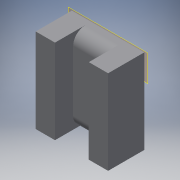
# Autodesk Inventor part: commutator_attachement_side_plate
Saved by Autodesk Inventor 2016 (Build 200138000, 138)
## iProperties
Created: 2016-09-28
Part Number: commutator_attachement_side_plate
Material: Generic
Document SubType Name: Modeling
Designer: ajar021
Density: 1 g/cm^3
Appearance: Default
Author: ajar021
Autodesk Inventor part; units mm, degrees
ref_plane "YZ Plane" through (0, 0, 0) normal (1, 0, 0) x (0, 1, 0)
ref_plane "XZ Plane" through (0, 0, 0) normal (0, 1, 0) x (-1, 0, 0)
ref_plane "XY Plane" through (0, 0, 0) normal (0, 0, 1) x (1, 0, 0)
ref_plane "Work Plane1" through (0, 0, 0) normal (0, 0, 1) x (1, 0, 0)
sketch "Sketch1" plane through (0, 0, 0) normal (0, 0, 1) x (1, 0, 0)
  line L0 (12, 0) -> (12, 4) projected
  line L1 (0, 4) -> (12, 4) projected
  line L2 (0, 0) -> (0, 4) projected
  line L3 (12, 0) -> (12, -10)
  line L4 (12, -10) -> (0, -10)
  line L5 (0, -10) -> (0, 4)
  line L6 (0, 4) -> (12, 4)
  line L7 (12, 4) -> (12, 0)
  dimension "d0" = 10
  constraints: 10 end point, 3 collinear, 1 perpendicular, 1 vertical
  measures "d0" distance of L0.start L3.end
extrude "Extrusion1" add sketch "Sketch1" along normal blind 3
sketch "Sketch2" plane through (0, 0, 3) normal (0, 0, 1) x (1, 0, 0)
  line L0 (12, -10) -> (12, 4) projected
  line L1 (12, 4) -> (0, 4) projected
  line L2 (0, 4) -> (0, -10) projected
  line L3 (0, -10) -> (12, -10) projected
  line L4 (6, 4) -> (8.8, 4)
  line L5 (6, 4) -> (3.2, 4)
  line L6 (8.8, 4) -> (8.8, -10)
  line L7 (8.8, -10) -> (12, -10)
  line L8 (12, 4) -> (8.8, 4)
  line L9 (3.2, 4) -> (3.2, -10)
  line L10 (3.2, -10) -> (0, -10)
  line L11 (0, -10) -> (0, 4)
  line L12 (0, 4) -> (3.2, 4)
  point P0 (0, 0)
  dimension "d3" = 2.8
  dimension "d4" = 2.8
  constraints: 18 end point, 4 collinear, 4 point on line, 3 perpendicular, 1 midpoint
  measures "d3" distance of L4.start L4.end
  measures "d4" distance of L5.end L4.start
extrude "Extrusion2" add sketch "Sketch2" along normal blind 3 contours L3 L6 L1 L0 | L3 L2 L1 L9
fillet "Fillet1" radius 2 1 edges at (6, 4, 3)
fillet "Fillet2" radius 2 1 edges at (6, -10, 3)
equation "\"d4\" = d3"
body "Solid1"
